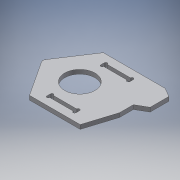
# Autodesk Inventor part: 胴体_サブフレーム_1_4
Saved by Autodesk Inventor 2018 (Build 220112000, 112)
## iProperties
Created: 2016-05-07
Part Number: 胴体_サブフレーム_1_4
Material: アルミニウム 2014-T4
Document SubType Name: Modeling
Designer: hiroaki
Density: 2.8 g/cm^3
Appearance: サテン
Mass: 10.894 g
Surface Area: 49.6118 cm^2
Volume: 3.89073 cm^3
Author: hiroaki
Autodesk Inventor part; units mm, degrees
ref_plane "YZ Plane" through (0, 0, 0) normal (1, 0, 0) x (0, 1, 0)
ref_plane "XZ Plane" through (0, 0, 0) normal (0, 1, 0) x (-1, 0, 0)
ref_plane "XY Plane" through (0, 0, 0) normal (0, 0, 1) x (1, 0, 0)
derived "胴体_基礎_1_3.ipt"
sketch "スケッチ1" plane through (0, 0, 0) normal (0, 0, 1) x (1, 0, 0)
  circle A0 centre (-13, 0) radius 1.55 construction
  circle A1 centre (13, 0) radius 1.55 construction
  line L0 (0, 0) -> (0, -11.5097) construction
  line L1 (-24, 57.0251) -> (-24, -5) construction
  line L2 (-24, -5) -> (28, -5) construction
  line L3 (-24, 57.0251) -> (-30.5, 72.9658) construction
  line L4 (-30.5, 72.9658) -> (-30.5, 112.7596) construction
  line L5 (-30.5, 112.7596) -> (-15, 120.25) construction
  line L6 (-15, 120.25) -> (28, 120.25) construction
  circle A2 centre (-3, 92) radius 11 projected
  line L7 (-15, 102.583) -> (-15, 81.417) construction
  line L8 (-3, 108) -> (36.5, 108) construction
  line L9 (36.5, 108) -> (36.5, 76) construction
  line L10 (36.5, 76) -> (-3, 76) construction
  arc A3 (-3, 108) -> (-15, 102.583) centre (-3, 92) ccw construction
  arc A4 (-15, 81.417) -> (-3, 76) centre (-3, 92) ccw construction
  line L11 (28, -5) -> (28, 73.75) construction
  line L12 (28, 73.75) -> (28, 120.25) construction
  line L13 (-2, 105.5) -> (25, 105.5) construction
  line L14 (25, 105.5) -> (25, 78.5) construction
  line L15 (25, 78.5) -> (-2, 78.5) construction
  line L16 (-2, 78.5) -> (-2, 105.5) construction
  circle A5 centre (-2, 105.5) radius 1.35 projected
  circle A6 centre (25, 105.5) radius 1.35 projected
  circle A7 centre (25, 78.5) radius 1.35 projected
  circle A8 centre (-2, 78.5) radius 1.35 projected
  circle A9 centre (-3, 92) radius 5.05 construction
  line L17 (-15, 110.25) -> (36.5, 110.25) construction
  line L18 (36.5, 110.25) -> (36.5, 73.75) construction
  line L19 (36.5, 73.75) -> (-15, 73.75) construction
  line L20 (-15, 73.75) -> (-15, 110.25) construction
  circle A10 centre (21.25, 92) radius 1.2 projected
  circle A11 centre (-3, 116.25) radius 1.2 projected
  circle A12 centre (-27.25, 92) radius 1.2 construction
  circle A13 centre (-3, 67.75) radius 1.2 projected
  line L21 (-6, 115.25) -> (15, 115.25) construction
  line L22 (15, 115.25) -> (15, 110.25) construction
  line L23 (15, 110.25) -> (-6, 110.25) construction
  line L24 (-6, 110.25) -> (-6, 115.25) construction
  circle A14 centre (-11, 112.75) radius 1.55 projected
  circle A15 centre (20, 112.75) radius 1.55 projected
  circle A16 centre (-11, 112.75) radius 7.5 construction
  circle A17 centre (-11, 71.25) radius 1.55 projected
  circle A18 centre (20, 71.25) radius 1.55 projected
  line L25 (-15, 92) -> (36.5, 92) construction
  line L26 (-6, 73.75) -> (15, 73.75) construction
  line L27 (15, 73.75) -> (15, 68.75) construction
  line L28 (15, 68.75) -> (-6, 68.75) construction
  line L29 (-6, 68.75) -> (-6, 73.75) construction
  line L30 (-15, 115.25) -> (24, 115.25) construction
  line L31 (24, 115.25) -> (24, 110.25) construction
  line L32 (24, 110.25) -> (-15, 110.25) construction
  line L33 (-15, 110.25) -> (-15, 115.25) construction
  circle A19 centre (-27.25, 92) radius 1.2
  circle A20 centre (-3, 116.25) radius 1.2
  circle A21 centre (-3, 67.75) radius 1.2
  circle A22 centre (21.25, 92) radius 1.2
  line L34 (-6.05, 112.8) -> (15.05, 112.8)
  line L35 (15.05, 112.8) -> (15.05, 110.2)
  line L36 (15.05, 110.2) -> (-6.05, 110.2)
  line L37 (-6.05, 110.2) -> (-6.05, 112.8)
  circle A23 centre (-5, 112.8) radius 1.05
  circle A24 centre (-5, 110.2) radius 1.05
  circle A25 centre (14, 112.8) radius 1.05
  circle A26 centre (14, 110.2) radius 1.05
  line L38 (-6.05, 73.8) -> (15.05, 73.8)
  line L39 (15.05, 73.8) -> (15.05, 71.2)
  line L40 (15.05, 71.2) -> (-6.05, 71.2)
  line L41 (-6.05, 71.2) -> (-6.05, 73.8)
  circle A27 centre (-5, 73.8) radius 1.05
  circle A28 centre (-5, 71.2) radius 1.05
  circle A29 centre (14, 73.8) radius 1.05
  circle A30 centre (14, 71.2) radius 1.05
  circle A31 centre (-27.25, 92) radius 2.5 construction
  line L42 (-29.3409, 93.3705) -> (-12.7059, 118.75)
  line L43 (-12.7059, 118.75) -> (24, 118.75)
  line L44 (24, 118.75) -> (30.8012, 97)
  line L45 (30.8012, 97) -> (30.8012, 87)
  line L46 (30.8012, 87) -> (24, 65.25)
  line L47 (24, 65.25) -> (-12.7059, 65.25)
  line L48 (-12.7059, 65.25) -> (-29.3409, 90.6295)
  arc A32 (-29.3409, 93.3705) -> (-29.3409, 90.6295) centre (-27.25, 92) ccw
  circle A33 centre (-11, 112.75) radius 4 construction
  line L49 (87, 127.7437) -> (87, 52.2479) construction
  circle A34 centre (25, 105.5) radius 3 construction
  circle A35 centre (-20, 50) radius 1.55 projected
  circle A36 centre (-20, 20) radius 1.55 projected
  circle A37 centre (10, 35) radius 1.55 projected
  line L50 (-39.5, 5) -> (35.9852, 5) construction
  line L51 (35.9852, 5) -> (35.9852, -12.9857) construction
  line L52 (35.9852, -12.9857) -> (-39.5, -12.9857) construction
  line L53 (-39.5, -12.9857) -> (-39.5, 5) construction
  line L54 (-6, 112.75) -> (4.9747, 112.75) construction
  circle A38 centre (-19.5, 105.25) radius 1.55 projected
  circle A39 centre (-19.5, 78.75) radius 1.55 projected
  line L55 (-22, 99.5) -> (-17, 99.5) construction
  line L56 (-17, 99.5) -> (-17, 84.5) construction
  line L57 (-17, 84.5) -> (-22, 84.5) construction
  line L58 (-22, 84.5) -> (-22, 99.5) construction
  circle A40 centre (-19.5, 100.55) radius 1.05 construction
  circle A41 centre (-26.5, 110.25) radius 1.55 projected
  circle A42 centre (-26.5, 73.75) radius 1.55 projected
  circle A43 centre (-26.5, 110.25) radius 4 construction
  circle A44 centre (-26.5, 73.75) radius 4 construction
  circle A45 centre (0, 0) radius 1.55 projected
  circle A46 centre (30, 114.5) radius 1.55
  circle A47 centre (34.2262, 105.4369) radius 1.55
  line L59 (30, 114.5) -> (34.2262, 105.4369) construction
  line L60 (28.4123, 117.25) -> (31.5877, 117.25) construction
  line L61 (31.5877, 117.25) -> (33.1754, 114.5) construction
  line L62 (33.1754, 114.5) -> (31.5877, 111.75) construction
  line L63 (31.5877, 111.75) -> (28.4123, 111.75) construction
  line L64 (28.4123, 111.75) -> (26.8246, 114.5) construction
  line L65 (26.8246, 114.5) -> (28.4123, 117.25) construction
  line L66 (34.2262, 102.2615) -> (31.4762, 103.8492) construction
  line L67 (31.4762, 103.8492) -> (31.4762, 107.0246) construction
  line L68 (31.4762, 107.0246) -> (34.2262, 108.6123) construction
  line L69 (34.2262, 108.6123) -> (36.9762, 107.0246) construction
  line L70 (36.9762, 107.0246) -> (36.9762, 103.8492) construction
  line L71 (36.9762, 103.8492) -> (34.2262, 102.2615) construction
  line L72 (24, 118.75) -> (31.9896, 118.75)
  line L73 (31.9896, 118.75) -> (38.4762, 115.005)
  line L74 (38.4762, 115.005) -> (38.4762, 101.4312)
  line L75 (38.4762, 101.4312) -> (30.8012, 97)
  circle A48 centre (30, 114.5) radius 3.1754 construction
  circle A49 centre (30, 114.5) radius 4.6754 construction
  point P0 (25, 92)
  point P1 (-6, 112.75)
  point P2 (30.8012, 92)
  point P3 (-19.5, 99.5)
  dimension "d1" = 2.1
  dimension "d2" = 0.05
  dimension "d3" = 5
  dimension "d4" = 90
  dimension "d5" = 10
  dimension "d35" = 2.5
  dimension "d42" = 0.05
  dimension "d43" = 2.5
  dimension "d44" = 0.05
  dimension "d45" = 65
  dimension "d46" = 10
  dimension "d47" = 3.1
  dimension "d48" = 5.5
  dimension "d49" = 1.5
  dimension "d50" = 10
  dimension "d51" = 1.5
  dimension "d52" = 1.5
  constraints: 68 end point, 11 centre point, 11 coincident, 10 point on line, 8 horizontal alignment, 7 horizontal, 7 tangent, 5 equal radius, 5 vertical, 4 vertical alignment, 3 symmetric about line, 2 equal length, 2 midpoint, 2 parallel, 2 perpendicular, 2 point on circle, 48 other
  measures "d2" distance between parallel lines of L37 L24
  measures "d3" diameter of A31
  measures "d4" distance from line of L49 A4.centre
  measures "d5" distance of L44.end L45.end
  measures "d35" distance from line of L43 A11.centre
  measures "d42" distance between parallel lines of L38 L26
  measures "d43" distance between parallel lines of L23 L54
  measures "d44" distance between parallel lines of L34 L54
  measures "d45" angle of L8 L59
  measures "d46" distance of L59.start L59.end
  measures "d47" diameter of A46
  measures "d48" distance between parallel lines of L63 L60
  measures "d49" distance between parallel lines of L60 L43
  measures "d50" horizontal distance of L59.start A15.centre
  measures "d51" distance between parallel lines of L74 L70
extrude "押し出し1" add sketch "スケッチ1" along normal blind 3 contours L42 L43 L44 L45 L46 L47 L48 A32 | L72 L73 L74 L75 L44 | A38 | A39
sketch "スケッチ8" plane through (31.9896, 118.75, 0) normal (0, 0, -1) x (-1, 0, 0)
  circle A0 centre (1.9896, -4.25) radius 1.55 projected
  circle A1 centre (1.9896, -4.25) radius 1.55
  circle A2 centre (-2.2365, -13.3131) radius 1.55 projected
  circle A3 centre (-2.2365, -13.3131) radius 1.55
  circle A4 centre (6.9896, -13.25) radius 1.35 projected
  circle A5 centre (6.9896, -13.25) radius 1.35
  circle A6 centre (11.9896, -6) radius 1.55 projected
  circle A7 centre (11.9896, -6) radius 1.55
  circle A8 centre (34.9896, -2.5) radius 1.2 projected
  circle A9 centre (34.9896, -2.5) radius 1.2
  circle A10 centre (42.9896, -6) radius 1.55 projected
  circle A11 centre (42.9896, -6) radius 1.55
  circle A12 centre (33.9896, -13.25) radius 1.35 projected
  circle A13 centre (33.9896, -13.25) radius 1.35
  circle A14 centre (10.7396, -26.75) radius 1.2 projected
  circle A15 centre (10.7396, -26.75) radius 1.2
  circle A16 centre (6.9896, -40.25) radius 1.35 projected
  circle A17 centre (6.9896, -40.25) radius 1.35
  circle A18 centre (11.9896, -47.5) radius 1.55 projected
  circle A19 centre (11.9896, -47.5) radius 1.55
  circle A20 centre (42.9896, -47.5) radius 1.55 projected
  circle A21 centre (42.9896, -47.5) radius 1.55
  circle A22 centre (33.9896, -40.25) radius 1.35 projected
  circle A23 centre (33.9896, -40.25) radius 1.35
  circle A24 centre (59.2396, -26.75) radius 1.2 projected
  circle A25 centre (59.2396, -26.75) radius 1.2
  circle A26 centre (34.9896, -51) radius 1.2 projected
  circle A27 centre (34.9896, -51) radius 1.2
  point P0 (31.9896, -118.75)
  constraints: 14 centre point, 14 coincident
extrude "押し出し5" add sketch "スケッチ8" against normal up to surface (3 mm away)
